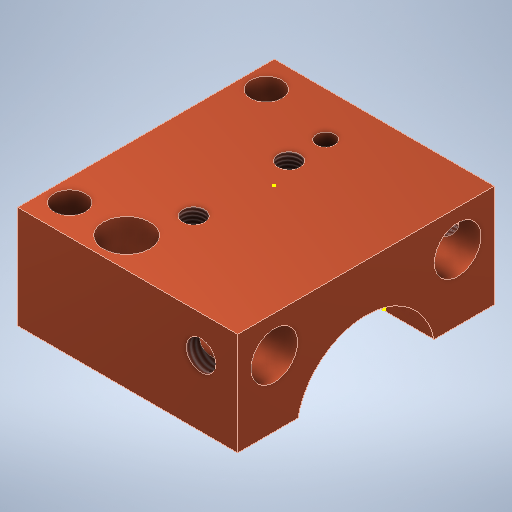
# Autodesk Inventor part: Rb oven housing top-back
Saved by Autodesk Inventor 2025.3 (Build 293356000, 356)
## iProperties
Created: 2025-04-11
Part Number: Rb oven housing top-back
Material: Copper
Document SubType Name: Modeling
Designer: E. Moreno
Density: 8.94 g/cm^3
Appearance: Copper - Polished
Author: E. Moreno
Title: Carcasa Horno - Superior
Autodesk Inventor part; units mm, degrees
ref_plane "YZ Plane" through (0, 0, 0) normal (1, 0, 0) x (0, 1, 0)
ref_plane "XZ Plane" through (0, 0, 0) normal (0, 1, 0) x (-1, 0, 0)
ref_plane "XY Plane" through (0, 0, 0) normal (0, 0, 1) x (1, 0, 0)
sketch "Sketch1" plane through (0, 0, 0) normal (0, 0, 1) x (1, 0, 0)
  line L0 (15, -7) -> (-15, -7)
  line L1 (-15, -7) -> (-15, 7)
  line L2 (-15, 7) -> (15, 7)
  line L3 (15, 7) -> (15, -7)
  line L4 (15, -7) -> (-15, 7) construction
  line L5 (-15, -7) -> (15, 7) construction
  point P0 (0, 0)
  dimension "d0" = 30
  dimension "d1" = 14
  constraints: 12 end point, 2 midpoint, 2 parallel, 1 horizontal, 1 perpendicular
  measures "d0" distance of L1.end L2.end
  measures "d1" distance of L0.end L1.end
extrude "Extrusion1" add sketch "Sketch1" along normal blind 35
sketch "Sketch3" plane through (15, -7, 0) normal (1, 0, 0) x (0, 0, -1)
  line L0 (0, 0) -> (-35, 0) projected
  line L1 (-17.5, 0) -> (-17.5, -2)
  arc A0 (-8.2129, 0) -> (-26.7871, 0) centre (-17.5, -2) ccw
  point P0 (0, 7)
  dimension "d4" = 2
  dimension "d5" = 19
  constraints: 2 end point, 2 point on circle, 2 point on line, 1 centre point, 1 coincident, 1 midpoint, 1 vertical
  measures "d4" distance of L1.start L1.end
  measures "d5" diameter of A0
extrude "Extrusion2" cut sketch "Sketch3" against normal blind 25
sketch "Sketch5" plane through (-15, 7, 0) normal (0, 1, 0) x (1, 0, 0)
  line L0 (30, 0) -> (0, 0) projected
  line L1 (30, -35) -> (0, -35) projected
  line L2 (0, -35) -> (0, -30.9)
  line L3 (0, 0) -> (0, -35) projected
  line L4 (0, -30.9) -> (2.75, -30.9)
  circle A0 centre (2.75, -30.9) radius 2
  line L5 (0, 0) -> (0, -4.1)
  line L6 (0, -4.1) -> (2.75, -4.1)
  circle A1 centre (2.75, -4.1) radius 2
  line L7 (2.75, -30.9) -> (10.75, -30.9)
  circle A2 centre (10.75, -30.9) radius 3.175
  point P0 (15, 0)
  dimension "d11" = 4.1
  dimension "d12" = 2.75
  dimension "d13" = 4
  dimension "d14" = 4.1
  dimension "d15" = 2.75
  dimension "d16" = 4
  dimension "d17" = 8
  dimension "d18" = 6.35
  constraints: 10 end point, 3 centre point, 3 coincident, 2 perpendicular, 2 point on line, 1 horizontal
  measures "d11" distance of L1.end L2.end
  measures "d12" distance of L2.end L4.end
  measures "d13" diameter of A0
  measures "d14" distance of L0.end L5.end
  measures "d15" distance of L5.end L6.end
  measures "d16" diameter of A1
  measures "d17" distance of L7.start L7.end
  measures "d18" diameter of A2
extrude "Extrusion3" cut sketch "Sketch5" against normal blind 100 contours A2
sketch "Sketch6" plane through (-15, 7, 0) normal (0, 1, 0) x (1, 0, 0)
  point P0 (15, 0)
sketch "Sketch7" plane through (15, -7, 0) normal (1, 0, 0) x (0, 0, -1)
  line L0 (0, 14) -> (-35, 14) projected
  line L1 (-35, 14) -> (-30, 14)
  line L2 (-30, 14) -> (-30, 9)
  line L3 (0, 14) -> (0, 0) projected
  line L4 (0, 14) -> (-5, 14)
  line L5 (-5, 14) -> (-5, 9)
  circle A0 centre (-30, 9) radius 3.175
  circle A1 centre (-5, 9) radius 3.175
  point P0 (0, 7)
  dimension "d21" = 5
  dimension "d22" = 5
  dimension "d23" = 5
  dimension "d24" = 5
  dimension "d25" = 6.35
  dimension "d26" = 6.35
  constraints: 8 end point, 2 centre point, 2 coincident, 2 point on line, 1 perpendicular, 1 vertical
  measures "d21" distance of L0.end L1.end
  measures "d22" distance of L1.end L2.end
  measures "d23" distance of L0.start L4.end
  measures "d24" distance of L4.end L5.end
  measures "d25" diameter of A0
  measures "d26" diameter of A1
extrude "Extrusion4" cut sketch "Sketch7" against normal blind 15
move or copy body "Move Body1" bodies to move or copy 1 copy no translate (-20, 0, 0)
move or copy body "Move Body2" bodies to move or copy 1 copy no translate (-5, 0, 0)
sketch "Sketch8" plane through (0, 0, 0) normal (1, 0, 0) x (0, 1, 0)
  point P0 (0, 0)
sketch "Sketch9" plane through (-40, 7, 0) normal (0, 1, 0) x (1, 0, 0)
  line L0 (30, -35) -> (0, -35) projected
  line L1 (0, -35) -> (0, -30.9)
  line L2 (0, 0) -> (0, -35) projected
  line L3 (0, -30.9) -> (3, -30.9)
  circle A0 centre (3, -30.9) radius 2.15
  line L4 (0, 0) -> (0, -4.1)
  line L5 (0, -4.1) -> (3, -4.1)
  circle A1 centre (3, -4.1) radius 2.15
  point P0 (40, 0)
  dimension "d35" = 4.1
  dimension "d36" = 3
  dimension "d37" = 4.3
  dimension "d38" = 4.1
  dimension "d39" = 4.3
  dimension "d40" = 3
  constraints: 8 end point, 2 centre point, 2 coincident, 2 perpendicular, 2 point on line
  measures "d35" distance of L0.end L1.end
  measures "d36" distance of L1.end L3.end
  measures "d37" diameter of A0
  measures "d38" distance of L2.start L4.end
  measures "d39" diameter of A1
  measures "d40" distance of L4.end L5.end
extrude "Extrusion5" cut sketch "Sketch9" against normal blind 14
sketch "Sketch14" plane through (-40, 7, 35) normal (0, 0, 1) x (1, 0, 0)
  line L0 (30, 0) -> (0, 0) projected
  line L1 (30, 0) -> (25, 0)
  line L2 (25, 0) -> (25, -5)
  circle A0 centre (25, -5) radius 2
  point P0 (40, -7)
  dimension "d47" = 5
  dimension "d48" = 5
  dimension "d49" = 4
  constraints: 4 end point, 1 centre point, 1 coincident, 1 perpendicular, 1 point on line
  measures "d47" distance of L0.start L1.end
  measures "d48" distance of L1.end L2.end
  measures "d49" diameter of A0
extrude "Extrusion6" cut sketch "Sketch14" against normal blind 3
sketch "Sketch15" plane through (-10, 7, 0) normal (0, 0, -1) x (-1, 0, 0)
  line L0 (0, -14) -> (0, 0) projected
  line L1 (0, 0) -> (5, 0)
  line L2 (0, 0) -> (30, 0) projected
  line L3 (5, 0) -> (5, -5)
  circle A0 centre (5, -5) radius 2
  point P0 (-10, -7)
  dimension "d52" = 5
  dimension "d53" = 5
  dimension "d54" = 4
  constraints: 4 end point, 1 centre point, 1 coincident, 1 perpendicular, 1 point on line
  measures "d52" distance of L0.end L1.end
  measures "d53" distance of L1.end L3.end
  measures "d54" diameter of A0
extrude "Extrusion7" cut sketch "Sketch15" against normal blind 4
thread "Thread3" size "M4x0.7" class "6H" standard "ANSI Metric M Profile" full length
thread "Thread4" size "M4x0.7" class "6H" standard "ANSI Metric M Profile" full length
sketch "Sketch16" plane through (-40, -7, 0) normal (-1, 0, 0) x (0, 0, 1)
  line L0 (0, 14) -> (35, 14) projected
  line L1 (0, 14) -> (17.5, 14)
  line L2 (17.5, 14) -> (17.5, -2)
  circle A0 centre (17.5, -2) radius 7.5
  point P0 (0, 7)
  dimension "d61" = 16
  dimension "d62" = 15
  constraints: 4 end point, 1 centre point, 1 coincident, 1 midpoint, 1 perpendicular
  measures "d61" distance of L1.end L2.end
  measures "d62" diameter of A0
extrude "Extrusion8" cut sketch "Sketch16" against normal blind 15
move or copy body "Move Body3" bodies to move or copy 1 copy no translate (25, 0, 0)
move or copy body "Move Body4" bodies to move or copy 1 copy no translate (10, 0, -15)
move or copy body "Move Body5" bodies to move or copy 1 copy no translate (-10, 0, 0)
sketch "Sketch17" plane through (15, -7, -15) normal (1, 0, 0) x (0, 0, -1)
  point P0 (-15, 7)
sketch "Sketch19" plane through (-15, 7, -15) normal (0, 1, 0) x (1, 0, 0)
  line L0 (30, 0) -> (0, 0) projected
  line L1 (0, 0) -> (0, -6)
  line L2 (0, 0) -> (6, 0) construction
  line L3 (0, -6) -> (13, -6)
  circle A0 centre (13, -6) radius 1.25
  line L4 (13, -6) -> (13, -8.5)
  line L5 (13, -6) -> (15.5, -6) construction
  point P0 (15, -15)
  dimension "d74" = 6
  dimension "d75" = 90
  dimension "d76" = 13
  dimension "d77" = 90
  dimension "d78" = 2.5
  dimension "d84" = 2.5
  dimension "d85" = 90
  constraints: 10 end point, 3 perpendicular, 2 horizontal, 2 vertical, 1 centre point, 1 coincident
  measures "d74" distance of L0.end L1.end
  measures "d75" angle of L1 L2
  measures "d76" distance of L1.end L3.end
  measures "d77" angle of L3 L1
  measures "d78" diameter of A0
  measures "d84" distance of L4.start L4.end
  measures "d85" angle of L4 L5
extrude "Extrusion9" cut sketch "Sketch19" against normal blind 13
sketch "Sketch20" plane through (-15, 7, -15) normal (0, 1, 0) x (1, 0, 0)
  circle A0 centre (13, -6) radius 1.25 projected
  line L0 (13, -6) -> (13, -11)
  circle A1 centre (13, -11) radius 1.5
  line L1 (30, 0) -> (0, 0) projected
  line L2 (13, -11) -> (26, -11) construction
  line L3 (0, 0) -> (0, -35) projected
  line L4 (0, -17.5) -> (30, -17.5)
  line L5 (30, -8.2129) -> (30, -26.7871) projected
  circle A2 centre (13, -24) radius 1.5
  point P0 (15, -15)
  dimension "d86" = 5
  dimension "d87" = 3
  constraints: 6 end point, 2 centre point, 2 midpoint, 1 coincident, 1 horizontal, 1 symmetric about line, 1 vertical, 1 other
  measures "d86" distance of L0.start L0.end
  measures "d87" diameter of A1
extrude "Extrusion10" cut sketch "Sketch20" against normal blind 6 contours A1 | A2
thread "Thread5" size "M3x0.5" class "6H" standard "ANSI Metric M Profile" full length
thread "Thread6" size "M3x0.5" class "6H" standard "ANSI Metric M Profile" full length
equation "\"d55\" = d54"
body "Solid1"
